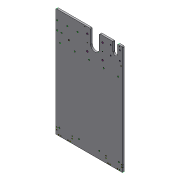
# Autodesk Inventor part: TL20240701-10110CV-002
Saved by Autodesk Inventor 2022.5 (Build 265521000, 521)
## iProperties
Category: DRIVE UNIT ASSY
Manager: 호상태
Company: 현대 트랜시스(대유)
Created: 2023-01-19
Part Number: TL20240701-10110CV-002
Project: SW PJT
Checked By: 김형민
Engr Approved By: 김시현
User Status: 1/1 x18
Material: SS400
Description: 0
Document SubType Name: Modeling
Mfg Approved By: 호상태
Designer: 박성규
Stock Number: 002
Mass: 13148.3 g
Surface Area: 1560.92 cm^2
Volume: 1670.68 cm^3
Density: 7.85 g/cm^3
Appearance: Painting-RAL7035
DETAIL: Coveryor Assembly
M/C TITLE: MEa/NEa차종 시트조립라인
SPECIFICATION: TL20221201-000000CV-005
DocNumber: 221118_Standard_v1
Folder: .\
VDS_Category: 엔지니어링
Detail Description: Processed products
Title: SIDE PLATE
Subject: SW차종 시트조립라인
Author: 박성규
Revision Number: A
Autodesk Inventor part; units mm, degrees
ref_plane "YZ Plane" through (0, 0, 0) normal (1, 0, 0) x (0, 1, 0)
ref_plane "XZ Plane" through (0, 0, 0) normal (0, 1, 0) x (-1, 0, 0)
ref_plane "XY Plane" through (0, 0, 0) normal (0, 0, 1) x (1, 0, 0)
sketch "스케치22" plane through (0, 0, 0) normal (0, 0, 1) x (1, 0, 0)
  line L0 (-230, 375) -> (230, 375)
  line L1 (230, 375) -> (230, -375)
  line L2 (230, -375) -> (-230, -375)
  line L3 (-230, -375) -> (-230, 375)
  line L4 (-230, 375) -> (230, -375) construction
  line L5 (230, 375) -> (-230, -375) construction
  point P0 (0, 0)
  dimension "d122" = 460
  dimension "HIGHT" = 750
  constraints: 12 end point, 2 midpoint, 2 parallel, 1 horizontal, 1 perpendicular
  measures "d122" distance of L0.start L0.end
  measures "HIGHT" distance of L0.end L1.end
extrude "돌출12" add sketch "스케치22" along normal blind 12
sketch "스케치25" plane through (0, 0, 0) normal (0, 0, -1) x (-1, 0, 0)
  line L0 (-230, 375) -> (230, 375) construction
  line L1 (-230, -375) -> (-230, 375) construction
  line L2 (-180, 314) -> (-180, 414) construction
  line L3 (-164, 314) -> (-164, 414)
  line L4 (-196, 414) -> (-196, 314)
  arc A0 (-196, 314) -> (-164, 314) centre (-180, 314) ccw
  arc A1 (-164, 414) -> (-196, 414) centre (-180, 414) ccw
  point P0 (0, 0)
  point P1 (-180, 364)
  dimension "d162" = 50
  dimension "d163" = 61
  dimension "d164" = 100
  dimension "d165" = 32
  constraints: 8 end point, 4 point on circle, 4 tangent, 2 centre point, 1 midpoint, 1 parallel, 1 vertical
  measures "d162" distance between parallel lines of L1 L2
  measures "d163" distance from line of L0 L2.start
  measures "d164" distance of L2.start L2.end
  measures "d165" distance between parallel lines of L3 L4
extrude "돌출13" cut sketch "스케치25" against normal through all
sketch "스케치38" plane through (0, 0, 0) normal (0, 0, -1) x (-1, 0, 0)
  line L0 (-40, 279.35) -> (-40, 431.2387) construction
  line L1 (-70, 279.35) -> (-70, 431.2387)
  line L2 (-10, 431.2387) -> (-10, 279.35)
  arc A0 (-70, 279.35) -> (-10, 279.35) centre (-40, 279.35) ccw
  arc A1 (-10, 431.2387) -> (-70, 431.2387) centre (-40, 431.2387) ccw
  line L3 (-230, -375) -> (-230, 375) projected
  line L4 (-230, 375) -> (-196, 375) projected
  point P0 (0, 0)
  point P1 (-40, 355.2944)
  point P2 (-230, 385)
  point P3 (-10, 355.2944)
  point P4 (-70, 355.2944)
  point P5 (-162, 390)
  point P6 (225, 390)
  point P7 (-10, 390)
  point P8 (-70, 390)
  dimension "d270" = 190
  dimension "d271" = 60
  dimension "d272" = 95.65
  constraints: 8 end point, 4 point on circle, 4 tangent, 3 midpoint, 2 centre point, 1 parallel, 1 vertical, 1 other
  measures "d270" distance from line of point (-40, 355.294) L3
  measures "d271" distance of point (-10, 355.294) point (-70, 355.294)
extrude "돌출19" cut sketch "스케치38" along normal through all both and the other way through all
sketch "스케치24" plane through (0, 0, 12) normal (0, 0, 1) x (1, 0, 0)
  line L0 (230, 375) -> (-230, 375) construction
  line L1 (-230, 375) -> (-230, -375) construction
  line L2 (230, -375) -> (230, 375) construction
  line L3 (-230, -375) -> (230, -375) projected
  point P0 (0, 0)
  point P1 (-200, 183)
  point P2 (-100, 183)
  point P3 (0, 183)
  point P4 (100, 183)
  point P5 (200, 183)
  point P6 (-110, -357)
  point P7 (-55, -357)
  point P8 (0, -357)
  point P9 (55, -357)
  point P10 (110, -357)
  dimension "d141" = 30
  dimension "d142" = 192
  dimension "d143" = 100
  dimension "d144" = 100
  dimension "d145" = 100
  dimension "d146" = 100
  dimension "d182" = 120
  dimension "d183" = 55
  dimension "d184" = 55
  dimension "d185" = 55
  dimension "d256" = 55
  dimension "d257" = 120
  dimension "d325" = 18
  constraints: 8 horizontal alignment
  measures "d141" distance from line of L1 point (-200, 183)
  measures "d142" distance from line of L0 point (-200, 183)
  measures "d143" distance of point (-100, 183) point (-200, 183)
  measures "d144" distance of point (0, 183) point (-100, 183)
  measures "d145" distance of point (0, 183) point (100, 183)
  measures "d146" distance of point (200, 183) point (100, 183)
  measures "d182" distance from line of L1 point (-110, -357)
  measures "d183" distance of point (-55, -357) point (-110, -357)
  measures "d184" distance of point (0, -357) point (-55, -357)
  measures "d185" distance of point (55, -357) point (0, -357)
  measures "d256" distance of point (110, -357) point (55, -357)
  measures "d257" distance from line of L2 point (110, -357)
  measures "d325" distance from line of point (-110, -357) L3
hole "구멍8" at (-200, 183, 12) at (-100, 183, 12) at (0, 183, 12) at (100, 183, 12) at (200, 183, 12) direction (0, 0, -1) diameter 9 end through all clearance for "Socket Head Cap Screw" size "M8" standard "TS Profile"
sketch "스케치23" plane through (0, 0, 12) normal (0, 0, 1) x (1, 0, 0)
  line L0 (230, 375) -> (-230, 375) construction
  line L1 (-230, 375) -> (-230, -375) construction
  line L2 (-230, -375) -> (230, -375) projected
  point P0 (0, 0)
  point P1 (-220, 309)
  point P2 (-220, 249)
  point P3 (-190, 249)
  point P4 (-150, 309)
  point P5 (-80, 309)
  point P6 (-220, -231)
  point P7 (-150, -231)
  point P8 (-80, -231)
  point P9 (-220, -291)
  point P10 (-190, -291)
  dimension "d126" = 66
  dimension "d128" = 126
  dimension "d129" = 10
  dimension "d130" = 10
  dimension "d131" = 70
  dimension "d132" = 70
  dimension "d133" = 30
  dimension "d154" = 10
  dimension "d155" = 30
  dimension "d158" = 10
  dimension "d159" = 70
  dimension "d160" = 70
  dimension "d323" = 84
  dimension "d324" = 144
  constraints: 6 horizontal alignment
  measures "d126" distance from line of L0 point (-220, 309)
  measures "d128" distance from line of L0 point (-220, 249)
  measures "d129" distance from line of L1 point (-220, 309)
  measures "d130" distance from line of L1 point (-220, 249)
  measures "d131" distance of point (-150, 309) point (-220, 309)
  measures "d132" distance of point (-80, 309) point (-150, 309)
  measures "d133" distance of point (-190, 249) point (-220, 249)
  measures "d154" distance from line of L1 point (-220, -291)
  measures "d155" distance of point (-220, -291) point (-190, -291)
  measures "d158" distance from line of L1 point (-220, -231)
  measures "d159" distance of point (-150, -231) point (-220, -231)
  measures "d160" distance of point (-80, -231) point (-150, -231)
  measures "d323" distance from line of point (-220, -291) L2
  measures "d324" distance from line of point (-220, -231) L2
hole "구멍7" at (-220, 309, 12) at (-220, 249, 12) at (-190, 249, 12) at (-150, 309, 12) at (-80, 309, 12) direction (0, 0, -1) diameter 9 end through all clearance for "Socket Head Cap Screw" size "M8" standard "TS Profile"
sketch "스케치26" plane through (0, 0, 0) normal (0, 0, -1) x (-1, 0, 0)
  arc A0 (-196, 314) -> (-164, 314) centre (-180, 314) ccw construction
  line L0 (-212, 282) -> (-148, 282) construction
  line L1 (-148, 282) -> (-148, 346) construction
  line L2 (-148, 346) -> (-212, 346) construction
  line L3 (-212, 346) -> (-212, 282) construction
  line L4 (-212, 282) -> (-148, 346) construction
  line L5 (-148, 282) -> (-212, 346) construction
  point P0 (0, 0)
  dimension "d168" = 64
  dimension "d169" = 64
  constraints: 12 end point, 4 coincident, 2 midpoint, 2 parallel, 1 horizontal, 1 perpendicular
  measures "d168" distance of L1.end L2.end
  measures "d169" distance of L0.end L1.end
hole "구멍9" at (212, 346, 0) at (212, 282, 0) at (148, 282, 0) at (148, 346, 0) direction (0, 0, 1) diameter 8.376 end through all thread size "M10x1.5" class "6H" standard "TS profile"
sketch "스케치27" plane through (0, 0, 0) normal (0, 0, -1) x (-1, 0, 0)
  line L0 (-230, -375) -> (-230, 375) projected
  line L1 (-230, 375) -> (-196, 375) projected
  line L2 (230, -375) -> (-230, -375) projected
  point P0 (0, 0)
  point P1 (-210, 367)
  point P2 (30, 367)
  point P3 (-210, -173)
  point P4 (30, -173)
  dimension "d326" = 20
  dimension "d327" = 240
  dimension "d328" = 8
  dimension "d329" = 202
  constraints: 2 horizontal alignment, 2 vertical alignment
  measures "d326" distance from line of point (-210, 367) L0
  measures "d327" distance of point (30, 367) point (-210, 367)
  measures "d328" distance from line of point (-210, 367) L1
  measures "d329" distance from line of point (-210, -173) L2
hole "구멍10" at (210, 367, 0) at (-30, 367, 0) direction (0, 0, 1) diameter 4.917 end through all thread size "M6x1" class "6H" standard "TS profile"
sketch "스케치28" plane through (0, 0, 12) normal (0, 0, 1) x (1, 0, 0)
  line L0 (164, 375) -> (-230, 375) construction
  line L1 (230, -375) -> (230, 375) projected
  point P0 (0, 0)
  point P1 (220, 256)
  dimension "d199" = 119
  dimension "d330" = 10
  measures "d199" distance from line of L0 point (220, 256)
  measures "d330" distance from line of L1 point (220, 256)
hole "구멍11" at (220, 256, 12) direction (0, 0, -1) diameter 6.6 end through all clearance for "Socket Head Cap Screw" size "M6" standard "TS Profile"
sketch "스케치37" plane through (0, 0, 12) normal (0, 0, 1) x (1, 0, 0)
  line L0 (230, -375) -> (230, 375) projected
  line L1 (-230, -375) -> (230, -375) projected
  point P0 (0, 0)
  point P1 (205, -325)
  point P2 (70, -325)
  point P3 (-70, -325)
  point P4 (-205, -325)
  point P5 (230, 385)
  dimension "d258" = 135
  dimension "d259" = 140
  dimension "d260" = 135
  dimension "d261" = 25
  dimension "d262" = 50
  constraints: 3 horizontal alignment
  measures "d258" distance of point (70, -325) point (205, -325)
  measures "d259" distance of point (-70, -325) point (70, -325)
  measures "d260" distance of point (-205, -325) point (-70, -325)
  measures "d261" distance from line of L0 point (205, -325)
  measures "d262" distance from line of L1 point (205, -325)
hole "구멍15" at (205, -325, 12) at (70, -325, 12) at (-70, -325, 12) at (-205, -325, 12) direction (0, 0, -1) diameter 9 end through all clearance for "Socket Head Cap Screw" size "M8" standard "TS Profile"
sketch "스케치39" plane through (0, 0, 0) normal (0, 0, -1) x (-1, 0, 0)
  line L0 (-230, -375) -> (-230, 375) projected
  arc A0 (-70, 279.35) -> (-10, 279.35) centre (-40, 279.35) ccw projected
  point P0 (0, 0)
  point P1 (-92.5, 331.85)
  point P2 (12.5, 331.85)
  point P3 (12.5, 226.85)
  point P4 (-92.5, 226.85)
  dimension "d332" = 105
  dimension "d333" = 105
  dimension "d334" = 52.5
  dimension "d335" = 52.5
  constraints: 2 horizontal alignment, 2 vertical alignment
  measures "d332" distance of point (12.5, 331.85) point (-92.5, 331.85)
  measures "d333" distance of point (-92.5, 226.85) point (-92.5, 331.85)
  measures "d334" horizontal distance of point (-92.5, 331.85) A0.centre
  measures "d335" horizontal distance of A0.centre point (-92.5, 331.85)
hole "구멍16" at (92.5, 331.85, 0) at (-12.5, 331.85, 0) at (-12.5, 226.85, 0) at (92.5, 226.85, 0) direction (0, 0, 1) diameter 11.835 end through all thread size "M14x2" class "6H" standard "TS profile"
sketch "스케치40" plane through (0, 0, 0) normal (0, 0, -1) x (-1, 0, 0)
  line L0 (-224, -331) -> (-116, -331)
  line L1 (-116, -331) -> (-116, -346)
  line L2 (-116, -346) -> (-224, -346)
  line L3 (-224, -346) -> (-224, -331)
  line L4 (-224, -331) -> (-116, -346) construction
  line L5 (-116, -331) -> (-224, -346) construction
  line L6 (-230, -375) -> (-230, 375) projected
  line L7 (230, -375) -> (-230, -375) projected
  point P0 (0, 0)
  point P1 (-210, -369)
  point P2 (-195, -369)
  point P3 (-145, -369)
  point P4 (-130, -369)
  point P5 (-170, -338.5)
  point P6 (-230, 385)
  dimension "d289" = 108
  dimension "d290" = 15
  dimension "d291" = 20
  dimension "d292" = 15
  dimension "d293" = 50
  dimension "d294" = 15
  dimension "d295" = 6
  dimension "d296" = 6
  dimension "d297" = 29
  constraints: 12 end point, 3 horizontal alignment, 2 midpoint, 2 parallel, 1 horizontal, 1 perpendicular
  measures "d289" distance of L1.end L2.end
  measures "d290" distance of L0.end L1.end
  measures "d291" distance from line of L6 point (-210, -369)
  measures "d292" distance of point (-195, -369) point (-210, -369)
  measures "d293" distance of point (-145, -369) point (-195, -369)
  measures "d294" distance of point (-130, -369) point (-145, -369)
  measures "d295" distance from line of L7 point (-210, -369)
  measures "d296" distance between parallel lines of L6 L3
  measures "d297" distance between parallel lines of L7 L2
hole "구멍17" at (210, -369, 0) at (195, -369, 0) at (145, -369, 0) at (130, -369, 0) at (224, -331, 0) at (224, -346, 0) at (116, -346, 0) at (116, -331, 0) direction (0, 0, 1) diameter 6.6 end through all counterbore diameter 11 counterbore depth 6.5 clearance for "Socket Head Cap Screw" size "M6" standard "TS Profile"
mirror "미러2" about plane through (0, 0, 0) normal (1, 0, 0) of "구멍17"
sketch "스케치41" plane through (0, 0, 12) normal (0, 0, 1) x (1, 0, 0)
  line L0 (10, 375) -> (-230, 375) projected
  line L1 (-230, 375) -> (-230, -375) projected
  point P0 (0, 0)
  point P1 (-139, 230.35)
  point P2 (5, 390)
  point P3 (-225, 390)
  point P4 (-230, 385)
  point P5 (10, 375)
  dimension "d312" = 144.65
  dimension "d313" = 91
  constraints: 1 other
  measures "d313" distance from line of L1 point (-139, 230.35)
hole "구멍18" at (-139, 230.35, 12) direction (0, 0, -1) diameter 10.106 end through all thread size "M12x1.75" class "6H" standard "TS profile"
sketch "Sketch42" plane through (0, 0, 12) normal (0, 0, 1) x (1, 0, 0)
  circle A0 centre (-12.5, 331.85) radius 5.9175 projected
  circle A1 centre (92.5, 226.85) radius 5.9175 projected
  point P0 (0, 0)
  point P1 (-12.5, 279.35)
  point P2 (92.5, 279.35)
  dimension "d314" = 105
  dimension "d315" = 52.5
  constraints: 2 vertical alignment, 1 horizontal alignment
  measures "d314" horizontal distance of A1.centre A0.centre
  measures "d315" distance of point (-12.5, 279.35) A0.centre
hole "Hole19" at (-12.5, 279.35, 12) at (92.5, 279.35, 12) direction (0, 0, -1) diameter 4.917 end through all thread size "M6x1" class "6H" standard "TS profile"
chamfer "Chamfer4" distance 5 angle 45 2 edges at (70, 375, 6) (10, 375, 6)
chamfer "Chamfer5" distance 2 angle 45 2 edges at (164, 375, 6) (196, 375, 6)
fillet "Fillet7" radius 5 2 edges at (-230, 375, 6) (230, 375, 6)
equation "\"d144\" = d143"
equation "\"d145\" = d143"
equation "\"d146\" = d143"
equation "\"d184\" = d183"
equation "\"d185\" = d184"
equation "\"d132\" = d131"
equation "\"d160\" = d159"
